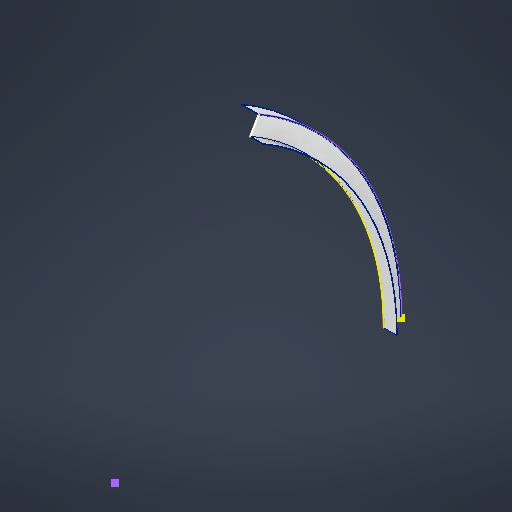
# Autodesk Inventor part: Support Ring Section, Z Section
Saved by Autodesk Inventor 2026.2 (Build 302298000, 298)
## iProperties
Created: 2026-01-30
Part Number: Support Ring Section, Z Section
Material: Aluminum 6061
Document SubType Name: Modeling
Designer: Lex Machina
Density: 2.7 g/cm^3
Appearance: Aluminum - Flat
Author: Lex Machina
Autodesk Inventor part; units mm, degrees
ref_plane "YZ Plane" through (0, 0, 0) normal (1, 0, 0) x (0, 1, 0)
ref_plane "XZ Plane" through (0, 0, 0) normal (0, 1, 0) x (-1, 0, 0)
ref_plane "XY Plane" through (0, 0, 0) normal (0, 0, 1) x (1, 0, 0)
sketch "Sketch1" plane through (0, 0, 0) normal (0, 1, 0) x (-1, 0, 0)
  line L0 (0, 0) -> (-130, 0)
  line L1 (-130, 0) -> (-130, -4)
  line L2 (-130, -4) -> (0, -4)
  line L3 (0, -4) -> (0, 0)
  line L4 (-130, -4) -> (-128.5, -4)
  line L5 (-128.5, -4) -> (-128.5, 126)
  line L6 (-128.5, 126) -> (-130, 126)
  line L7 (-130, 126) -> (-130, -4)
  line L8 (-128.5, 126) -> (-226, 126)
  line L9 (-226, 126) -> (-226, 122)
  line L10 (-226, 122) -> (-128.5, 122)
  line L11 (-128.5, 122) -> (-128.5, 126)
  line L12 (-65, -4) -> (-65, 2114)
  line L13 (-65, 2114) -> (-122.8585, 2114)
  point P0 (-128.5, 0)
  point P1 (-130, 122)
  dimension "d0" = 130
  dimension "d1" = 4
  dimension "d2" = 1.5
  dimension "d3" = 130
  dimension "d4" = 97.5
  dimension "d5" = 4
  dimension "d6" = 2118
  constraints: 28 end point, 6 parallel, 4 perpendicular, 3 horizontal, 1 midpoint, 1 vertical
  measures "d0" distance of L2.end L1.end
  measures "d1" distance of L1.end L0.end
  measures "d2" distance of L6.end L5.end
  measures "d3" distance of L5.end L4.end
  measures "d4" distance of L10.end L9.end
  measures "d5" distance of L9.end L8.end
  measures "d6" distance of L12.start L12.end
revolve "Revolution1" add sketch "Sketch1" angle 59.865 about axis through (65, 0, 2114) along (1, 0, 0)
sketch "Sketch2" plane through (130, 0, 122) normal (1, 0, 0) x (0, 0, -1)
  line L0 (-4, 0) -> (0, 0) projected
  arc A0 (-4, 0) -> (-993.9462, 1719.3117) centre (-1992, 0) ccw projected
  arc A1 (-4, 0) -> (-993.9462, 1719.3117) centre (-1992, 0) ccw
  line L1 (-930.6893, 1828.2821) -> (-993.9462, 1719.3117) projected
  line L2 (-928.6811, 1831.7415) -> (-930.6893, 1828.2821) projected
  line L3 (-993.9462, 1719.3117) -> (-928.6811, 1831.7415)
  line L4 (0, 0) -> (126, 0) projected
  arc A2 (126, 0) -> (-928.6811, 1831.7415) centre (-1992, 0) ccw
  point P0 (122, 0)
  constraints: 4 point on circle, 2 centre point, 2 end point, 1 collinear
body "Solid1"
